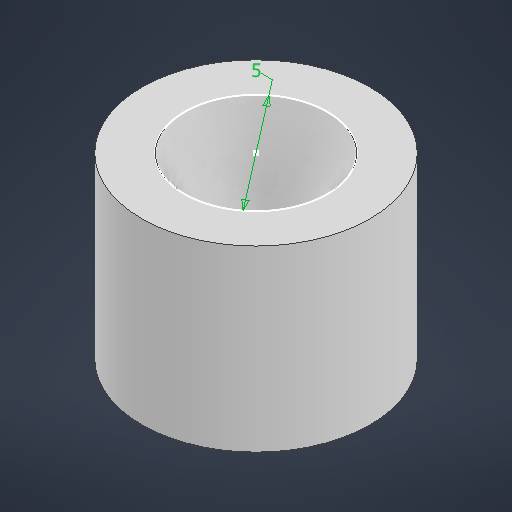
# Autodesk Inventor part: Acoustic Horn 30deg V1
Saved by Autodesk Inventor 2026 (Build 300175050, 175E)
## iProperties
Created: 2025-06-27
Part Number: Acoustic Horn 30deg V1
Material: Generic
Document SubType Name: Modeling
Designer: STW
Density: 1 g/cm^3
Appearance: Default
Author: STW
Autodesk Inventor part; units mm, degrees
ref_plane "YZ Plane" through (0, 0, 0) normal (1, 0, 0) x (0, 1, 0)
ref_plane "XZ Plane" through (0, 0, 0) normal (0, 1, 0) x (-1, 0, 0)
ref_plane "XY Plane" through (0, 0, 0) normal (0, 0, 1) x (1, 0, 0)
sketch "Sketch1" plane through (0, 0, 0) normal (0, 1, 0) x (-1, 0, 0)
  circle A0 centre (0, 0) radius 0.35
  circle A1 centre (0, 0) radius 4
  dimension "d0" = 0.7
  dimension "d2" = 8
  constraints: 2 centre point, 1 coincident, 1 concentric
  measures "d0" diameter of A0
  measures "d2" diameter of A1
extrude "Extrusion1" add sketch "Sketch1" along normal blind 6.26
sketch "Sketch2" plane through (0, 6.26, 0) normal (0, 1, 0) x (1, 0, 0)
  circle A0 centre (0, 0) radius 2.5
  dimension "d10" = 5
  constraints: 1 centre point, 1 coincident
  measures "d10" diameter of A0
sketch "Sketch3" plane through (0, 0, 0) normal (0, -1, 0) x (1, 0, 0)
  line L0 (-1.8, 1.8) -> (1.8, 1.8)
  line L1 (1.8, 1.8) -> (1.8, -1.8)
  line L2 (1.8, -1.8) -> (-1.8, -1.8)
  line L3 (-1.8, -1.8) -> (-1.8, 1.8)
  line L4 (-1.8, 1.8) -> (1.8, -1.8) construction
  line L5 (1.8, 1.8) -> (-1.8, -1.8) construction
  arc A0 (1.8, 1.6) -> (1.6, 1.8) centre (1.8, 1.8) ccw
  arc A1 (1.6, -1.8) -> (1.8, -1.6) centre (1.8, -1.8) ccw
  arc A2 (-1.8, -1.6) -> (-1.6, -1.8) centre (-1.8, -1.8) ccw
  arc A3 (-1.6, 1.8) -> (-1.8, 1.6) centre (-1.8, 1.8) ccw
  point P0 (0, 0)
  dimension "d11" = 0.2
  dimension "d12" = 3.6
  dimension "d13" = 3.6
  constraints: 12 end point, 8 point on circle, 8 point on line, 4 centre point, 4 coincident, 3 equal radius, 2 midpoint, 2 parallel, 1 horizontal, 1 perpendicular
  measures "d11" radius of A0
  measures "d12" distance of L0.end L1.end
  measures "d13" distance of L1.end L2.end
extrude "Extrusion2" cut sketch "Sketch3" against normal blind 1.27
sketch "Sketch5" plane through (0, 0, 0) normal (0, 0, 1) x (1, 0, 0)
  line L0 (-0.35, 1.27) -> (0.35, 1.27) projected
  line L1 (4, 6.26) -> (-4, 6.26) projected
  arc A0 (-0.35, 1.27) -> (-2.5, 6.26) centre (-11.8764, -0.7381) ccw
  line L2 (0, 1.27) -> (0, 6.26)
  line L3 (0.35, 1.27) -> (0, 1.27)
  line L4 (0.35, 6.26) -> (0.35, 1.27) projected
  line L5 (0.35, 6.26) -> (-2.5, 6.26)
  point P0 (0, 0)
  dimension "d17" = 2.5
  dimension "d23" = 11.7
  constraints: 6 end point, 3 point on line, 2 collinear, 2 midpoint, 2 point on circle, 1 centre point, 1 vertical
  measures "d17" distance of L2.end L5.end
  measures "d23" radius of A0
revolve "Revolution1" cut sketch "Sketch5" angle 360 about axis through (0, 1.27, 0) along (0, 1, 0) contours A0 L1 L2 L0
fillet "Fillet1" radius 0.1 1 edges at (0.35, 1.27, 0)
body "Solid1"
